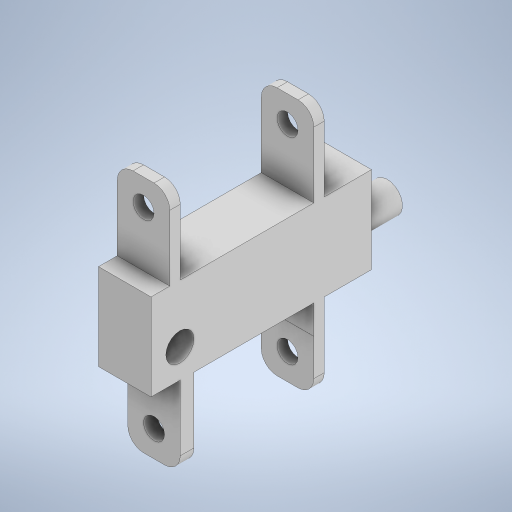
# Autodesk Inventor part: DudukanRodaDepan
Saved by Autodesk Inventor 2024 (Build 280153000, 153)
## iProperties
Created: 2025-12-11
Part Number: DudukanRodaDepan
Material: Generic
Document SubType Name: Modeling
Designer: risda
Density: 1 g/cm^3
Appearance: Default
Author: risda
Autodesk Inventor part; units mm, degrees
ref_plane "YZ Plane" through (0, 0, 0) normal (1, 0, 0) x (0, 1, 0)
ref_plane "XZ Plane" through (0, 0, 0) normal (0, 1, 0) x (-1, 0, 0)
ref_plane "XY Plane" through (0, 0, 0) normal (0, 0, 1) x (1, 0, 0)
sketch "Sketch1" plane through (0, 0, 0) normal (0, 1, 0) x (-1, 0, 0)
  line L0 (0, 0) -> (0, -15)
  line L1 (0, -15) -> (-10, -15)
  line L2 (-10, -15) -> (-10, 0)
  line L3 (-10, 0) -> (0, 0)
  dimension "d0" = 15
  dimension "d1" = 10
  constraints: 8 end point, 2 perpendicular, 2 vertical
  measures "d0" distance of L0.start L0.end
  measures "d1" distance of L0.end L1.end
extrude "Extrusion1" add sketch "Sketch1" along normal blind 22
sketch "Sketch3" plane through (10, 0, -15) normal (0, 0, -1) x (-1, 0, 0)
  line L0 (0, 0) -> (0, 22) projected
  line L1 (0, 11) -> (5, 11)
  circle A0 centre (5, 11) radius 2.9
  point P0 (10, 0)
  dimension "d9" = 5
  dimension "d10" = 5.8
  constraints: 2 end point, 1 centre point, 1 coincident, 1 horizontal, 1 midpoint
  measures "d9" distance of L1.start L1.end
  measures "d10" diameter of A0
extrude "Extrusion3" add sketch "Sketch3" along normal blind 8
sketch "Sketch4" plane through (0, 0, 0) normal (0, -1, 0) x (1, 0, 0)
  line L0 (0, 0) -> (0, -6)
  line L1 (0, -15) -> (0, 0) projected
  line L2 (0, -6) -> (10, -6)
  line L3 (10, -6.8) -> (0, -6.8) projected
  line L4 (10, -6) -> (10, -4)
  line L5 (10, -4) -> (0, -4)
  dimension "d13" = 6
  dimension "d14" = 2
  constraints: 8 end point, 2 perpendicular, 2 point on line, 1 parallel
  measures "d13" distance of L0.start L0.end
  measures "d14" distance of L2.end L4.end
extrude "Extrusion4" add sketch "Sketch4" along normal blind 10
fillet "Fillet1" radius 3 2 edges at (10, -10, -5) (0, -10, -5)
sketch "Sketch5" plane through (10, 0, -6) normal (0, 0, -1) x (-1, 0, 0)
  line L0 (0, 0) -> (5, 0)
  line L1 (0, 0) -> (10, 0) projected
  line L2 (5, 0) -> (5, -5)
  circle A0 centre (5, -5) radius 2
  dimension "d18" = 5
  dimension "d19" = 5
  dimension "d20" = 4
  constraints: 4 end point, 1 centre point, 1 coincident, 1 midpoint, 1 perpendicular
  measures "d18" distance of L0.start L0.end
  measures "d19" distance of L0.end L2.end
  measures "d20" diameter of A0
extrude "Extrusion5" cut sketch "Sketch5" against normal blind 10
sketch "Sketch6" plane through (0, 0, 0) normal (0, -1, 0) x (1, 0, 0)
  line L0 (10, -6) -> (10, -15) projected
  line L1 (10, -15) -> (10, -6)
  line L2 (10, -6) -> (0, -6)
  line L3 (0, -6) -> (0, -15)
  line L4 (0, -15) -> (10, -15)
  line L5 (0, 0) -> (10, 0) projected
  line L6 (10, -4.0095) -> (0, -4.0095)
  line L7 (0, -4.0095) -> (0, 0)
  line L8 (0, 0) -> (10, 0)
  line L9 (10, 0) -> (10, -4.0095)
  constraints: 16 end point, 4 perpendicular, 3 equal length, 1 horizontal
extrude "Extrusion6" cut sketch "Sketch6" against normal blind 5.5
sketch "Sketch7" plane through (0, 22, 0) normal (0, 0, 1) x (1, 0, 0)
  line L0 (10, -16.5) -> (10, 0) projected
  line L1 (10, 0) -> (0, 0)
  line L2 (0, 0) -> (0, -16.5)
  line L3 (0, -16.5) -> (10, -16.5)
  line L4 (10, -16.5) -> (10, 0)
  point P0 (0, -22)
  constraints: 8 end point, 2 parallel, 1 horizontal, 1 perpendicular
extrude "Extrusion7" add sketch "Sketch7" along normal blind 27
sketch "Sketch8" plane through (10, -7, -4) normal (1, 0, 0) x (0, 0, -1)
  line L0 (11, 29) -> (-31, 29) projected
  line L1 (11, 29) -> (-25.5, 29)
  line L2 (-25.5, 29) -> (-25.5, 18)
  circle A0 centre (-25.5, 18) radius 2.675
  point P0 (-4, 7)
  dimension "d28" = 36.5
  dimension "d29" = 11
  dimension "d30" = 5.35
  constraints: 4 end point, 1 centre point, 1 coincident, 1 perpendicular, 1 point on line
  measures "d28" distance of L0.start L1.end
  measures "d29" distance of L1.end L2.end
  measures "d30" diameter of A0
extrude "Extrusion8" cut sketch "Sketch8" against normal blind 40
sketch "Sketch9" plane through (0, 22, 0) normal (0, 1, 0) x (1, 0, 0)
  line L0 (0, 15) -> (0, -27) projected
  line L1 (10, 15) -> (10, -27) projected
  line L2 (0, -23.4243) -> (10, -23.4243)
  line L3 (10, -23.4243) -> (10, -21.4243)
  line L4 (10, -21.4243) -> (0, -21.4243)
  line L5 (0, -21.4243) -> (0, -23.4243)
  point P0 (0, 0)
  point P1 (0, -21.4243)
  dimension "d33" = 2
  constraints: 8 end point, 2 parallel, 2 point on line, 1 horizontal, 1 perpendicular
  measures "d33" distance of L2.end L3.end
extrude "Extrusion9" add sketch "Sketch9" along normal blind 15.5
fillet "Fillet3" radius 3 2 edges at (10, 37.5, 22.4243) (0, 37.5, 22.4243)
sketch "Sketch10" plane through (10, 22, 21.4243) normal (0, 0, -1) x (-1, 0, 0)
  line L0 (7, 15.5) -> (3, 15.5) projected
  line L1 (5, 15.5) -> (5, 10.5)
  circle A0 centre (5, 10.5) radius 2
  point P0 (10, -22)
  dimension "d37" = 5
  dimension "d38" = 4
  constraints: 2 end point, 1 centre point, 1 coincident, 1 midpoint, 1 vertical
  measures "d37" distance of L1.start L1.end
  measures "d38" diameter of A0
extrude "Extrusion10" cut sketch "Sketch10" against normal blind 15.5
sketch "Sketch11" plane through (0, 22, 0) normal (0, 1, 0) x (1, 0, 0)
  line L0 (0, 6) -> (10, 6) projected
  line L1 (0, 4.0095) -> (10, 4.0095) projected
  line L2 (0, 6) -> (10, 6)
  line L3 (10, 6) -> (10, 4.0095)
  line L4 (10, 4.0095) -> (0, 4.0095)
  line L5 (0, 4.0095) -> (0, 6)
  point P0 (0, 0)
  constraints: 8 end point, 2 parallel, 1 horizontal, 1 perpendicular
extrude "Extrusion11" add sketch "Sketch11" along normal blind 15.5
fillet "Fillet4" radius 3 2 edges at (10, 37.5, -5.0048) (0, 37.5, -5.0048)
sketch "Sketch12" plane through (10, 22, -6) normal (0, 0, -1) x (-1, 0, 0)
  circle A0 centre (5, 10.5) radius 2 projected
  circle A1 centre (5, 10.5) radius 2
  point P0 (10, -22)
  constraints: 1 centre point, 1 coincident
extrude "Extrusion12" cut sketch "Sketch12" against normal blind 10
sketch "Sketch13" plane through (0, 5.5, 0) normal (0, -1, 0) x (1, 0, 0)
  line L0 (10, 18.825) -> (0, 18.825) projected
  line L1 (0, 21.4243) -> (10, 21.4243) projected
  line L2 (10, 18.825) -> (0, 18.825)
  line L3 (0, 18.825) -> (0, 21.4243)
  line L4 (0, 21.4243) -> (10, 21.4243)
  line L5 (10, 21.4243) -> (10, 18.825)
  point P0 (0, 0)
  constraints: 8 end point, 2 parallel, 1 horizontal, 1 perpendicular, 1 point on line
extrude "Extrusion13" add sketch "Sketch13" along normal blind 15.5
fillet "Fillet5" radius 3 2 edges at (0, -10, 20.1246) (10, -10, 20.1246)
sketch "Sketch14" plane through (0, 5.5, 21.4243) normal (0, 0, 1) x (1, 0, 0)
  circle A0 centre (5, -10.5) radius 2 projected
  circle A1 centre (5, -10.5) radius 2
  point P0 (0, -5.5)
  constraints: 1 centre point, 1 coincident
extrude "Extrusion14" cut sketch "Sketch14" against normal blind 15.5
body "Solid1"
